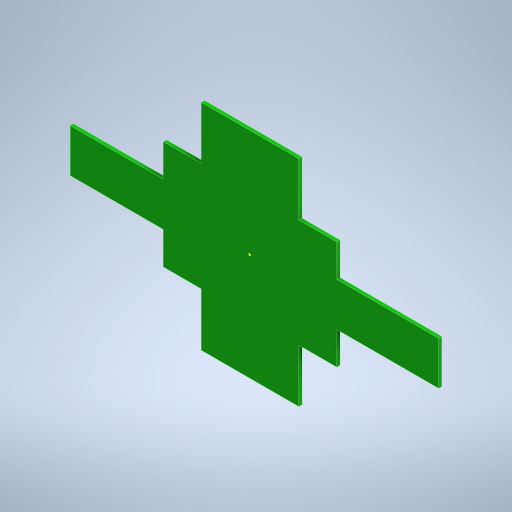
# Autodesk Inventor part: Platine
Saved by Autodesk Inventor 2024 (Build 280153000, 153)
## iProperties
Created: 2024-05-15
Part Number: Platine
Material: Generisch
Document SubType Name: Modeling
Designer: month
Density: 1 g/cm^3
Appearance: Dunkelgrün
Author: month
Autodesk Inventor part; units mm, degrees
ref_plane "YZ Plane" through (0, 0, 0) normal (1, 0, 0) x (0, 1, 0)
ref_plane "XZ Plane" through (0, 0, 0) normal (0, 1, 0) x (-1, 0, 0)
ref_plane "XY Plane" through (0, 0, 0) normal (0, 0, 1) x (1, 0, 0)
sketch "Skizze1" plane through (0, 0, 0) normal (0, 1, 0) x (-1, 0, 0)
  point P0 (0, 0)
sketch "Skizze2" plane through (0, 0, 0) normal (0, 1, 0) x (-1, 0, 0)
  line L0 (0, 99) -> (45, 99)
  line L1 (45, 99) -> (45, 50)
  line L2 (45, 50) -> (80, 50)
  line L3 (80, 50) -> (80, 20)
  line L4 (80, 20) -> (166.0252, 20)
  line L5 (166.0252, 20) -> (166.0252, -20)
  line L6 (166.0252, -20) -> (80, -20)
  line L7 (80, -20) -> (80, -50)
  line L8 (80, -50) -> (45, -50)
  line L9 (45, -50) -> (45, -99)
  line L10 (45, -99) -> (-45, -99)
  line L11 (-45, -99) -> (-45, -50)
  line L12 (-45, -50) -> (-80, -50)
  line L13 (-80, -50) -> (-80, -20)
  line L14 (-80, -20) -> (-173.9748, -20)
  line L15 (-173.9748, -20) -> (-173.9748, 20)
  line L16 (-173.9748, 20) -> (-80, 20)
  line L17 (-80, 20) -> (-80, 50)
  line L18 (-80, 50) -> (-45, 50)
  line L19 (-45, 50) -> (-45, 99)
  line L20 (-45, 99) -> (0, 99)
  line L21 (166.0252, 0) -> (-173.9748, 0)
  line L22 (0, 99) -> (0, -99)
  point P0 (0, 0)
  point P1 (-62.5, -50)
  point P2 (-62.5, 50)
  point P3 (0, -99)
  point P4 (-80, -35)
  point P5 (80, -35)
  dimension "d0" = 340
  dimension "d1" = 40
  dimension "d2" = 100
  dimension "d3" = 198
  dimension "d4" = 160
  dimension "d5" = 90
  dimension "d6" = 86.0252
  constraints: 46 end point, 17 perpendicular, 10 point on line, 9 midpoint, 2 horizontal, 9 other
  measures "d0" distance of L21.start L21.end
  measures "d1" distance of L14.end L15.end
  measures "d2" distance of point (-62.5, -50) point (-62.5, 50)
  measures "d3" distance from line of point (0, -99) L0
  measures "d4" distance of point (-80, -35) point (80, -35)
  measures "d5" distance between parallel lines of L11 L9
  measures "d6" distance of L5.end L6.end
extrude "Extrusion1" add sketch "Skizze2" along normal blind 3
